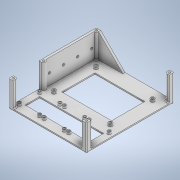
# Autodesk Inventor part: controlBoardCase
Saved by Autodesk Inventor 2020 (Build 240168000, 168)
## iProperties
Created: 2021-04-26
Part Number: controlBoardCase
Material: Generic
Document SubType Name: Modeling
Designer: PAB
Density: 1 g/cm^3
Appearance: Default
Author: PAB
Autodesk Inventor part; units mm, degrees
ref_plane "YZ Plane" through (0, 0, 0) normal (1, 0, 0) x (0, 1, 0)
ref_plane "XZ Plane" through (0, 0, 0) normal (0, 1, 0) x (-1, 0, 0)
ref_plane "XY Plane" through (0, 0, 0) normal (0, 0, 1) x (1, 0, 0)
sketch "Sketch1" plane through (0, 0, 0) normal (0, 1, 0) x (-1, 0, 0)
  line L0 (70, 57.5) -> (-70, 57.5)
  line L1 (-70, 57.5) -> (-70, -57.5)
  line L2 (-70, -57.5) -> (70, -57.5)
  line L3 (70, -57.5) -> (70, 57.5)
  point P0 (0, 0)
  dimension "d0" = 140
  dimension "d1" = 115
  constraints: 8 end point, 2 parallel, 1 horizontal, 1 perpendicular
  measures "d0" distance of L2.end L1.end
  measures "d1" distance of L1.end L0.end
extrude "Extrusion1" add sketch "Sketch1" along normal blind 4
sketch "Sketch2" plane through (0, 4, 0) normal (0, 1, 0) x (1, 0, 0)
  circle A0 centre (50.925, 38.05) radius 3.5
  circle A1 centre (-50.925, 38.05) radius 3.5
  circle A2 centre (-50.925, -38.05) radius 3.5
  circle A3 centre (50.925, -38.05) radius 3.5
  point P0 (0, 0)
  dimension "d4" = 7
  dimension "d5" = 7
  dimension "d6" = 7
  dimension "d7" = 7
  dimension "d8" = 38.05
  dimension "d9" = 76.1
  dimension "d10" = 38.05
  dimension "d11" = 76.1
  dimension "d12" = 50.925
  dimension "d13" = 101.85
  dimension "d14" = 50.925
  dimension "d15" = 101.85
  constraints: 4 centre point
  measures "d4" diameter of A0
  measures "d5" diameter of A1
  measures "d6" diameter of A2
  measures "d7" diameter of A3
  measures "d8" vertical distance of A0.centre point (0, 0)
  measures "d9" distance of A3.centre A0.centre
  measures "d10" vertical distance of point (0, 0) A1.centre
  measures "d11" distance of A2.centre A1.centre
  measures "d12" horizontal distance of point (0, 0) A2.centre
  measures "d13" distance of A2.centre A3.centre
  measures "d14" horizontal distance of A1.centre point (0, 0)
  measures "d15" distance of A0.centre A1.centre
extrude "Extrusion2" add sketch "Sketch2" along normal blind 4
sketch "Sketch3" plane through (-50.925, 8, -38.05) normal (0, 1, 0) x (1, 0, 0)
  circle A0 centre (0, 0) radius 3.5 projected
  circle A1 centre (0, 0) radius 2
  circle A2 centre (101.85, 0) radius 3.5 projected
  circle A3 centre (101.85, 0) radius 2
  circle A4 centre (101.85, -76.1) radius 3.5 projected
  circle A5 centre (101.85, -76.1) radius 2
  circle A6 centre (0, -76.1) radius 3.5 projected
  circle A7 centre (0, -76.1) radius 2
  point P0 (50.925, -38.05)
  dimension "d18" = 4
  dimension "d19" = 4
  dimension "d20" = 4
  dimension "d21" = 4
  constraints: 4 centre point, 4 coincident
  measures "d18" diameter of A1
  measures "d19" diameter of A3
  measures "d20" diameter of A5
  measures "d21" diameter of A7
extrude "Extrusion3" cut sketch "Sketch3" against normal blind 20 contours A1 | A3 | A5 | A7
sketch "Sketch4" plane through (-70, 0, 57.5) normal (0, 0, 1) x (1, 0, 0)
  line L0 (0, 0) -> (0, 4) projected
  line L1 (140, 4) -> (0, 4) projected
  line L2 (0, 0) -> (140, 0)
  line L3 (140, 0) -> (140, 4)
  line L4 (140, 4) -> (0, 4)
  line L5 (0, 4) -> (0, 0)
  point P0 (70, 0)
  constraints: 8 end point, 2 parallel, 1 horizontal, 1 perpendicular
extrude "Extrusion4" add sketch "Sketch4" along normal blind 42.8625
sketch "Sketch6" plane through (0, 4, 0) normal (0, 1, 0) x (1, 0, 0)
  circle A0 centre (-18.256, -52) radius 3
  circle A1 centre (-18.256, -88.512) radius 3
  circle A2 centre (-26.256, -52) radius 3
  circle A3 centre (-62.768, -52) radius 3
  circle A4 centre (-26.256, -88.512) radius 3
  circle A5 centre (-62.768, -88.512) radius 3
  point P0 (0, 0)
  dimension "d31" = 6
  dimension "d32" = 6
  dimension "d34" = 6
  dimension "d35" = 6
  dimension "d36" = 6
  dimension "d37" = 6
  constraints: 6 centre point
  measures "d31" diameter of A0
  measures "d32" diameter of A1
  measures "d34" diameter of A2
  measures "d35" diameter of A3
  measures "d36" diameter of A4
  measures "d37" diameter of A5
extrude "Extrusion5" add sketch "Sketch6" along normal blind 4
sketch "Sketch7" plane through (-18.256, 8, 52) normal (0, 1, 0) x (1, 0, 0)
  circle A0 centre (0, 0) radius 3 projected
  circle A1 centre (0, 0) radius 2
  circle A2 centre (-8, 0) radius 3 projected
  circle A3 centre (-8, 0) radius 2
  circle A4 centre (-44.512, 0) radius 3 projected
  circle A5 centre (-44.512, 0) radius 2
  circle A6 centre (-44.512, -36.512) radius 3 projected
  circle A7 centre (-44.512, -36.512) radius 2
  circle A8 centre (-8, -36.512) radius 3 projected
  circle A9 centre (-8, -36.512) radius 2
  circle A10 centre (0, -36.512) radius 3 projected
  circle A11 centre (0, -36.512) radius 2
  point P0 (18.256, 52)
  dimension "d40" = 4
  dimension "d41" = 4
  dimension "d42" = 4
  dimension "d43" = 4
  dimension "d44" = 4
  dimension "d45" = 4
  constraints: 6 centre point, 6 coincident
  measures "d40" diameter of A1
  measures "d41" diameter of A3
  measures "d42" diameter of A5
  measures "d43" diameter of A7
  measures "d44" diameter of A9
  measures "d45" diameter of A11
extrude "Extrusion6" cut sketch "Sketch7" against normal blind 20 contours A1 | A3 | A5 | A7 | A9 | A11
mirror "Mirror1" about plane through (0, 0, 0) normal (1, 0, 0) of "Extrusion6", "Extrusion5"
sketch "Sketch8" plane through (0, 4, 0) normal (0, 1, 0) x (1, 0, 0)
  line L0 (-45, -30) -> (45, -30)
  line L1 (45, -30) -> (45, 30)
  line L2 (45, 30) -> (-45, 30)
  line L3 (-45, 30) -> (-45, -30)
  line L4 (-57.768, -57) -> (57.768, -57)
  line L5 (57.768, -57) -> (57.768, -83.512)
  line L6 (57.768, -83.512) -> (-57.768, -83.512)
  line L7 (-57.768, -83.512) -> (-57.768, -57)
  point P0 (0, 0)
  dimension "d48" = 90
  dimension "d49" = 60
  dimension "d50" = 115.536
  dimension "d51" = 26.512
  constraints: 16 end point, 4 parallel, 2 horizontal, 2 perpendicular
  measures "d48" distance of L2.end L1.end
  measures "d49" distance of L1.end L0.end
  measures "d50" distance of L5.end L6.end
  measures "d51" distance of L4.end L5.end
extrude "Extrusion7" cut sketch "Sketch8" against normal blind 20
sketch "Sketch9" plane through (0, 4, 0) normal (0, 1, 0) x (1, 0, 0)
  line L0 (70, -100.3625) -> (-70, -100.3625) projected
  line L1 (-70, -100.3625) -> (-62, -100.3625)
  line L2 (-62, -100.3625) -> (-62, -92.3625)
  line L3 (-62, -92.3625) -> (-70, -92.3625)
  line L4 (-70, -92.3625) -> (-70, -100.3625)
  line L5 (70, -100.3625) -> (62, -100.3625)
  line L6 (62, -100.3625) -> (62, -92.3625)
  line L7 (62, -92.3625) -> (70, -92.3625)
  line L8 (70, -92.3625) -> (70, -100.3625)
  line L9 (70, 57.5) -> (70, -100.3625) projected
  line L10 (70, 57.5) -> (62, 57.5)
  line L11 (62, 57.5) -> (62, 49.5)
  line L12 (62, 49.5) -> (70, 49.5)
  line L13 (70, 49.5) -> (70, 57.5)
  line L14 (70, 57.5) -> (-70, 57.5) projected
  line L15 (-70, 57.5) -> (-62, 57.5)
  line L16 (-62, 57.5) -> (-62, 49.5)
  line L17 (-62, 49.5) -> (-70, 49.5)
  line L18 (-70, 49.5) -> (-70, 57.5)
  point P0 (0, 0)
  dimension "d54" = 8
  dimension "d55" = 8
  dimension "d56" = 8
  dimension "d57" = 8
  dimension "d58" = 8
  dimension "d59" = 8
  dimension "d60" = 8
  dimension "d61" = 8
  dimension "d100" = 0
  constraints: 32 end point, 8 parallel, 4 horizontal, 4 perpendicular, 1 point on line
  measures "d54" distance of L3.end L2.end
  measures "d55" distance of L2.end L1.end
  measures "d56" distance of L6.end L7.end
  measures "d57" distance of L5.end L6.end
  measures "d58" distance of L12.end L11.end
  measures "d59" distance of L11.end L10.end
  measures "d60" distance of L16.end L17.end
  measures "d61" distance of L15.end L16.end
  measures "d100" distance between parallel lines of L9 L8
extrude "Extrusion8" add sketch "Sketch9" along normal blind 44
fillet "Fillet1" radius 4 4 edges at (-62, 26, 92.3625) (-62, 26, -49.5) (62, 26, -49.5) (62, 26, 92.3625)
sketch "Sketch10" plane through (0, 48, 0) normal (0, 1, 0) x (1, 0, 0)
  arc A0 (-62, -96.3625) -> (-66, -92.3625) centre (-66, -96.3625) ccw projected
  circle A1 centre (-66, -96.3625) radius 2
  arc A2 (-66, 49.5) -> (-62, 53.5) centre (-66, 53.5) ccw projected
  circle A3 centre (-66, 53.5) radius 2
  arc A4 (62, 53.5) -> (66, 49.5) centre (66, 53.5) ccw projected
  circle A5 centre (66, 53.5) radius 2
  arc A6 (66, -92.3625) -> (62, -96.3625) centre (66, -96.3625) ccw projected
  circle A7 centre (66, -96.3625) radius 2
  point P0 (0, 0)
  dimension "d65" = 4
  dimension "d66" = 4
  dimension "d67" = 4
  dimension "d68" = 4
  constraints: 4 centre point, 4 coincident
  measures "d65" diameter of A1
  measures "d66" diameter of A3
  measures "d67" diameter of A5
  measures "d68" diameter of A7
extrude "Extrusion9" cut sketch "Sketch10" against normal blind 60
fillet "Fillet2" radius 2 12 edges at (-62, 4, -55.5) (-68, 4, -49.5) (-63.1716, 4, -50.6716) (-63.1716, 4, 93.5341) (-68, 4, 92.3625) (-62, 4, 98.3625) (63.1716, 4, -50.6716) (62, 4, -55.5) (68, 4, -49.5) (63.1716, 4, 93.5341) (62, 4, 98.3625) (68, 4, 92.3625)
sketch "Sketch11" plane through (0, 4, 0) normal (0, 1, 0) x (1, 0, 0)
  line L0 (-66, 49.5) -> (-70, 49.5) projected
  line L1 (-70, 49.5) -> (-66, 49.5)
  line L2 (-66, 49.5) -> (-66, -45.5)
  line L3 (-66, -45.5) -> (-70, -45.5)
  line L4 (-70, -45.5) -> (-70, 49.5)
  point P0 (0, 0)
  dimension "d72" = 4
  dimension "d73" = 95
  constraints: 8 end point, 2 parallel, 1 horizontal, 1 perpendicular
  measures "d72" distance of L2.end L3.end
  measures "d73" distance of L1.end L2.end
extrude "Extrusion10" add sketch "Sketch11" along normal blind 44
sketch "Sketch12" plane through (-70, 0, -57.5) normal (-1, 0, 0) x (0, 0, 1)
  circle A0 centre (12.7, 24) radius 4.325
  circle A1 centre (38.1, 24) radius 4.325
  circle A2 centre (63.5, 24) radius 4.325
  circle A3 centre (88.9, 24) radius 4.325
  point P0 (57.5, 0)
  dimension "d76" = 8.65
  dimension "d77" = 8.65
  dimension "d78" = 8.65
  dimension "d79" = 8.65
  constraints: 4 centre point
  measures "d76" diameter of A0
  measures "d77" diameter of A1
  measures "d78" diameter of A2
  measures "d79" diameter of A3
extrude "Extrusion11" add sketch "Sketch12" along normal blind 5
chamfer "Chamfer1" distance 1.5 angle 45 4 edges at (-75, 24, -49.125) (-75, 24, -23.725) (-75, 24, 1.675) (-75, 24, 27.075)
sketch "Sketch13" plane through (0, 4, 0) normal (0, 1, 0) x (1, 0, 0)
  line L0 (-70, -45.5) -> (-66, -45.5) projected
  line L1 (-70, -45.5) -> (-62, -45.5)
  line L2 (-62, -45.5) -> (-62, -37.5)
  line L3 (-62, -37.5) -> (-70, -37.5)
  line L4 (-70, -37.5) -> (-70, -45.5)
  point P0 (0, 0)
  dimension "d86" = 8
  dimension "d87" = 8
  constraints: 8 end point, 2 parallel, 1 horizontal, 1 perpendicular
  measures "d86" distance of L3.end L2.end
  measures "d87" distance of L2.end L1.end
extrude "Extrusion12" add sketch "Sketch13" along normal blind 44
fillet "Fillet4" radius 4 2 edges at (-62, 26, 45.5) (-62, 26, 37.5)
sketch "Sketch14" plane through (0, 48, 0) normal (0, 1, 0) x (1, 0, 0)
  arc A0 (-66, -45.5) -> (-66, -37.5) centre (-66, -41.5) ccw projected
  circle A1 centre (-66, -41.5) radius 2
  point P0 (0, 0)
  dimension "d91" = 4
  constraints: 1 centre point, 1 coincident
  measures "d91" diameter of A1
extrude "Extrusion13" cut sketch "Sketch14" against normal blind 60
sketch "Sketch15" plane through (-75, 24, -44.8) normal (-1, 0, 0) x (0, 0, 1)
  circle A0 centre (0, 0) radius 2
  circle A1 centre (25.4, 0) radius 2
  circle A2 centre (50.8, 0) radius 4.325 projected
  circle A3 centre (50.8, 0) radius 2
  circle A4 centre (76.2, 0) radius 4.325 projected
  circle A5 centre (76.2, 0) radius 2
  point P0 (44.8, -24)
  dimension "d94" = 4
  dimension "d95" = 4
  dimension "d96" = 4
  dimension "d97" = 4
  constraints: 4 centre point, 2 coincident
  measures "d94" diameter of A0
  measures "d95" diameter of A1
  measures "d96" diameter of A3
  measures "d97" diameter of A5
extrude "Extrusion14" cut sketch "Sketch15" against normal blind 15 contours A0 | A1 | A3 | A5
sketch "Sketch16" plane through (0, 4, 0) normal (0, 1, 0) x (1, 0, 0)
  line L0 (-62, 57.5) -> (-62, 53.5) projected
  line L1 (-62, 57.5) -> (-18, 57.5)
  line L2 (-18, 57.5) -> (-18, 53.5)
  line L3 (-18, 53.5) -> (-62, 53.5)
  line L4 (-62, 53.5) -> (-62, 57.5)
  point P0 (0, 0)
  dimension "d101" = 44
  dimension "d102" = 4
  constraints: 8 end point, 2 parallel, 1 horizontal, 1 perpendicular
  measures "d101" distance of L2.end L3.end
  measures "d102" distance of L1.end L2.end
extrude "Extrusion15" add sketch "Sketch16" along normal blind 44
sketch "Sketch17" plane through (70, 0, -57.5) normal (0, 0, -1) x (-1, 0, 0)
  line L0 (88, 48) -> (140, 48) projected
  line L1 (132, 48) -> (132, 6) projected
  line L2 (88, 48) -> (132, 48)
  line L3 (88, 4) -> (88, 48) projected
  line L4 (132, 48) -> (88, 4)
  line L5 (88, 4) -> (88, 48)
  point P0 (70, 0)
  constraints: 6 end point, 1 collinear, 1 perpendicular
extrude "Extrusion16" cut sketch "Sketch17" against normal blind 44
fillet "Fillet5" radius 2 16 edges at (0, 0, -57.5) (70, 0, 21.4312) (0, 0, 100.3625) (-70, 0, 21.4312) (70, 24, 100.3625) (70, 24, -57.5) (-70, 24, 100.3625) (-70, 24, -57.5) (0, 0, 83.512) (-57.768, 0, 70.256) (0, 0, 57) (57.768, 0, 70.256) (0, 0, 30) (-45, 0, 0) (0, 0, -30) (45, 0, 0)
body "Solid1"
